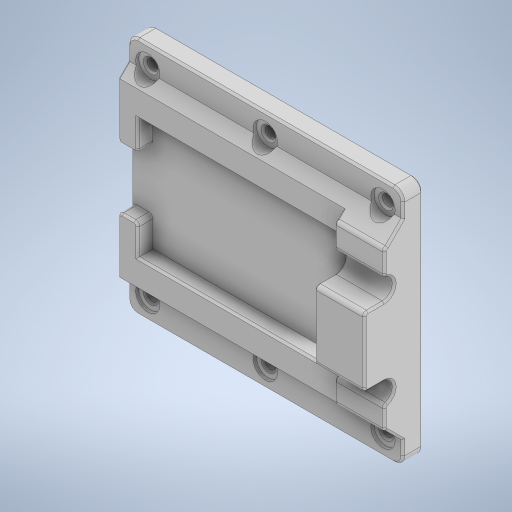
# Autodesk Inventor part: X-Idler Jig v0.1
Saved by Autodesk Inventor 2023 (Build 270158000, 158)
## iProperties
Created: 2023-07-27
Part Number: X-Idler Jig v0.1
Material: Generic
Document SubType Name: Modeling
Designer: Parker
Density: 1 g/cm^3
Appearance: Default
Author: Parker
Autodesk Inventor part; units mm, degrees
ref_plane "YZ Plane" through (0, 0, 0) normal (1, 0, 0) x (0, 1, 0)
sketch "Sketch1" plane through (0, 0, 0) normal (0, 0, 1) x (1, 0, 0)
  line L0 (-286, 0.5) -> (-242, 0.5) projected
  line L1 (-286, 60.5) -> (-286, 0.5) projected
  line L2 (-286, 60.5) -> (-242, 60.5) projected
  line L3 (-242, 60.5) -> (-242, 38.2446) projected
  line L4 (-242, 26.7554) -> (-242, 0.5) projected
  line L5 (-241.8, 60.7) -> (-286.2, 60.7)
  line L6 (-286.2, 60.7) -> (-286.2, 0.3)
  line L7 (-286.2, 0.3) -> (-241.8, 0.3)
  line L8 (-241.8, 0.3) -> (-241.8, 21.75)
  arc A0 (-241.8, 21.75) -> (-248, 27.95) centre (-248, 21.75) ccw
  arc A1 (-248, 37.05) -> (-248, 27.95) centre (-248, 32.5) ccw
  arc A2 (-248, 37.05) -> (-241.8, 43.25) centre (-248, 43.25) ccw
  line L9 (-241.8, 43.25) -> (-241.8, 60.7)
  line L10 (-185, -9.7) -> (-160, -9.7)
  line L11 (-160, -9.7) -> (-160, 70.7)
  line L12 (-160, 70.7) -> (-185, 70.7)
  line L13 (-185, 70.7) -> (-185, -9.7)
  line L14 (238, 2.5) -> (-240, 2.5)
  line L15 (238, 57.5) -> (-240, 57.5)
  line L16 (-185, 60.7) -> (-288.2, 60.7)
  line L17 (-288.2, 60.7) -> (-288.2, 0.3)
  line L18 (-288.2, 0.3) -> (-185, 0.3)
  line L19 (-185, 0.3) -> (-185, 60.7)
  line L20 (-185, -9.7) -> (-298.2, -9.7)
  line L21 (-298.2, -9.7) -> (-298.2, 70.7)
  line L22 (-298.2, 70.7) -> (-185, 70.7)
  line L23 (-185, 70.7) -> (-185, -9.7)
  line L24 (-278.2, 15.5) -> (-298.2, 15.5)
  line L25 (-298.2, 15.5) -> (-298.2, 45.5)
  line L26 (-298.2, 45.5) -> (-278.2, 45.5)
  line L27 (-278.2, 45.5) -> (-278.2, 15.5)
  line L28 (-278.2, 15.5) -> (-298.2, 45.5) construction
  line L29 (-298.2, 15.5) -> (-278.2, 45.5) construction
  arc A3 (-243.7143, 34.962) -> (-242, 38.2446) centre (-246, 38.2446) ccw projected
  arc A4 (-243.7143, 34.962) -> (-243.7143, 30.038) centre (-242, 32.5) ccw projected
  arc A5 (-242, 26.7554) -> (-243.7143, 30.038) centre (-246, 26.7554) ccw projected
  point P0 (0, 0)
  point P1 (-172.5, 70.7)
  point P2 (-288.2, 30.5)
  point P3 (-288.2, 15.5)
  point P4 (-288.2, 45.5)
  dimension "d0" = 0.2
  dimension "d2" = 57
  dimension "d6" = 2
  dimension "d7" = 10
  dimension "d8" = 10
  dimension "d9" = 10
  dimension "d10" = 25
  dimension "d57" = 30
  constraints: 51 end point, 8 parallel, 6 horizontal, 6 point on circle, 4 midpoint, 4 perpendicular, 4 point on line, 3 centre point, 7 other
  measures "d0" distance between parallel lines of L2 L5
  measures "d2" distance between parallel lines of L4 L13
  measures "d6" distance between parallel lines of L17 L6
  measures "d7" distance between parallel lines of L18 L20
  measures "d8" distance between parallel lines of L16 L22
  measures "d9" distance between parallel lines of L21 L17
  measures "d10" distance of L10.start L10.end
  measures "d57" distance of L24.end L25.end
extrude "Extrusion1" add sketch "Sketch1" along normal blind 15 contours L7 L18 L13 L20 L21 L24 L17 | L16 L17 L26 L21 L22 L13 L5
sketch "Sketch2" plane through (0, 0, 0) normal (0, 0, 1) x (1, 0, 0)
  line L0 (-160, 70.7) -> (-185, 70.7) projected
  line L1 (-160, -9.7) -> (-160, 70.7) projected
  line L2 (-185, 70.7) -> (-185, -9.7) projected
  line L3 (-185, -9.7) -> (-160, -9.7) projected
  point P0 (0, 0)
extrude "Extrusion2" add sketch "Sketch2" along normal blind 19.5
ref_plane "Work Plane1" through (0, 0, 0) normal (0, 0, 1) x (1, 0, 0)
sketch "Sketch3" plane through (0, 0, 0) normal (0, 0, 1) x (1, 0, 0)
  line L0 (-160, 70.7) -> (-298.2, 70.7) projected
  line L1 (-160, 90.7) -> (-298.2, 90.7)
  line L2 (-298.2, 90.7) -> (-298.2, -29.7)
  line L3 (-298.2, -29.7) -> (-160, -29.7)
  line L4 (-160, -29.7) -> (-160, 90.7)
  line L5 (-298.2, -9.7) -> (-160, -9.7) projected
  point P0 (0, 0)
  point P1 (-229.1, -29.7)
  point P2 (-160, -9.7)
  dimension "d15" = 20
  dimension "d16" = 20
  constraints: 8 end point, 2 parallel, 2 point on line, 1 horizontal, 1 midpoint, 1 perpendicular
  measures "d15" distance between parallel lines of L0 L1
  measures "d16" distance from line of L5 point (-229.1, -29.7)
extrude "Extrusion3" add sketch "Sketch3" along normal blind 10 contours L0 L2 L1 L4 | L4 L3 L2 L5
ref_plane "Work Plane2" through (-286, 0.5, 7.5) normal (0, 0, -1) x (0, 1, 0)
extrude "Extrusion5" add sketch "Sketch3" along normal up to surface (7.5 mm away) contours L4 L5 L2 L0
sketch "Sketch4" plane through (0, 0, 10) normal (0, 0, 1) x (1, 0, 0)
  line L0 (-298.2, -9.7) -> (-160, -9.7) projected
  line L1 (-298.2, -9.7) -> (-298.2, -29.7) projected
  line L2 (-298.2, -29.7) -> (-160, -29.7) projected
  line L3 (-160, -29.7) -> (-160, -9.7) projected
  line L4 (-160, 70.7) -> (-298.2, 70.7) projected
  line L5 (-160, 70.7) -> (-160, 90.7) projected
  line L6 (-160, 90.7) -> (-298.2, 90.7) projected
  line L7 (-298.2, 90.7) -> (-298.2, 70.7) projected
  line L8 (-170, -19.7) -> (-288.2, -19.7)
  line L9 (-288.2, -19.7) -> (-288.2, 80.7)
  line L10 (-288.2, 80.7) -> (-170, 80.7)
  line L11 (-170, 80.7) -> (-170, -19.7)
  point P0 (0, 0)
  point P1 (-229.1, 80.7)
  point P2 (-229.1, -19.7)
  dimension "d19" = 10
  dimension "d20" = 10
  dimension "d21" = 10
  dimension "d22" = 10
  constraints: 8 end point, 4 coincident, 2 midpoint, 2 parallel, 1 horizontal, 1 perpendicular
  measures "d19" distance between parallel lines of L2 L8
  measures "d20" distance between parallel lines of L3 L11
  measures "d21" distance between parallel lines of L7 L9
  measures "d22" distance between parallel lines of L6 L10
hole "Hole1" at (-170, -19.7, 10) at (-288.2, -19.7, 10) at (-288.2, 80.7, 10) at (-170, 80.7, 10) at (-229.1, 80.7, 10) at (-229.1, -19.7, 10) direction (0, 0, -1) diameter 5.5 end through all counterbore diameter 12.24 counterbore depth 1.5 clearance for "Hex Head Bolt" size "M5" standard "Ansi Metric M Profile"
fillet "Fillet1" radius 5 4 edges at (-160, 90.7, 5) (-298.2, 90.7, 5) (-298.2, -29.7, 5) (-160, -29.7, 5)
chamfer "Chamfer1" distance 8 angle 45 2 edges at (-229.1, 70.7, 10) (-229.1, -9.7, 10)
sketch "Sketch5" plane through (-160, -9.7, 19.5) normal (1, 0, 0) x (0, 0, -1)
  circle A0 centre (0, 62.2) radius 5 projected
  circle A1 centre (0, 17.2) radius 5 projected
  circle A2 centre (0, 17.2) radius 5.1
  circle A3 centre (0, 62.2) radius 5.1
  point P0 (19.5, 9.7)
  dimension "d34" = 0.1
  dimension "d35" = 0.1
  constraints: 2 centre point
  measures "d34" radial gap between concentric circles of A1 A2
  measures "d35" radial gap between concentric circles of A0 A3
extrude "Extrusion4" cut sketch "Sketch5" against normal up to surface (25 mm away) contours A0 | A1 | A2 | A3
sketch "Sketch7" plane through (0, 0, 19.5) normal (0, 0, 1) x (1, 0, 0)
  line L0 (-160, 47.4) -> (-185, 47.4) projected
  line L1 (-185, 47.4) -> (-185, 12.6) projected
  line L2 (-185, 12.6) -> (-160, 12.6) projected
  line L3 (-160, 12.6) -> (-160, 47.4) projected
  point P0 (0, 0)
extrude "Extrusion7" add sketch "Sketch7" along normal blind 10
fillet "Fillet2" radius 2 6 edges at (-172.5, 57.6, 19.5) (-172.5, 70.7, 19.5) (-172.5, -9.7, 19.5) (-172.5, 2.4, 19.5) (-172.5, 47.4, 29.5) (-172.5, 12.6, 29.5)
chamfer "Chamfer2" distance 1 angle 45 20 edges at (-160, -3.538, 19.5) (-160, 1.8861, 19.1011) (-160, 8.2257, 14.4519) (-160, -8.9883, 19.0811) (-160, 64.038, 19.5) (-160, 69.9883, 19.0811) (-160, 58.1139, 19.1011) (-160, 51.7743, 14.4519) (-185, 64.038, 19.5) (-185, 58.1139, 19.1011) (-185, 51.7743, 14.4519) (-185, 69.9883, 19.0811) (-185, -3.538, 19.5) (-185, -8.9883, 19.0811) (-185, 1.8861, 19.1011) (-185, 8.2257, 14.4519) (-185, 72.2, 16.5) (-185, -11.2, 16.5) (-160, -13.7, 14) (-160, 74.7, 14)
chamfer "Chamfer3" distance 1 angle 45 6 edges at (-236.6, 0.3, 15) (-288.2, 7.9, 15) (-288.2, 53.1, 15) (-236.6, 60.7, 15) (-298.2, 1.4, 15) (-298.2, 59.6, 15)
chamfer "Chamfer4" distance 1 angle 45 31 edges at (-170, 83.45, 8.5) (-288.2, 83.45, 8.5) (-288.2, -16.95, 8.5) (-170, -16.95, 8.5) (-229.1, 90.7, 0) (-296.7355, 89.2355, 0) (-296.7355, -28.2355, 0) (-229.1, -29.7, 0) (-161.4645, -28.2355, 0) (-160, 30.5, 0) (-161.4645, 89.2355, 0) (-170, 83.45, 0) (-170, -16.95, 0) (-288.2, -16.95, 0) (-288.2, 83.45, 0) (-229.1, 90.7, 10) (-296.7355, 89.2355, 10) (-298.2, 82.2, 10) (-161.4645, 89.2355, 10) (-160, 77.9929, 10) (-160, 82.2, 10) (-160, -16.9929, 10) (-160, -21.2, 10) (-161.4645, -28.2355, 10) (-229.1, -29.7, 10) (-296.7355, -28.2355, 10) (-298.2, -21.2, 10) (-229.1, -16.95, 8.5) (-229.1, -16.95, 0) (-229.1, 83.45, 0) (-229.1, 83.45, 8.5)
chamfer "Chamfer5" distance 1 angle 45 4 edges at (-298.2, 79.2, 9.5) (-298.2, 76.7, 12) (-298.2, -18.2, 9.5) (-298.2, -15.7, 12)
fillet "Fillet3" radius 2 4 edges at (-298.2, 45.5, 10.75) (-288.2, 45.5, 10.75) (-298.2, 15.5, 10.75) (-288.2, 15.5, 10.75)
chamfer "Chamfer6" distance 1 angle 45 6 edges at (-293.2, 15.5, 15) (-296.7176, 15.4319, 15) (-289.6824, 15.4319, 15) (-293.2, 45.5, 15) (-289.6824, 45.5681, 15) (-296.7176, 45.5681, 15)
body "Solid1"
